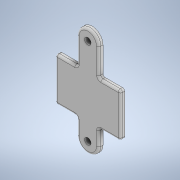
# Autodesk Inventor part: joy_mount_T
Saved by Autodesk Inventor 2021.4 (Build 254397000, 397)
## iProperties
Created: 2023-11-22
Part Number: joy_mount_T
Material: 一般
Document SubType Name: Modeling
Designer: ryusei
Density: 1 g/cm^3
Appearance: 既定
Author: ryusei
Autodesk Inventor part; units mm, degrees
ref_plane "YZ Plane" through (0, 0, 0) normal (1, 0, 0) x (0, 1, 0)
ref_plane "XZ Plane" through (0, 0, 0) normal (0, 1, 0) x (-1, 0, 0)
ref_plane "XY Plane" through (0, 0, 0) normal (0, 0, 1) x (1, 0, 0)
sketch "スケッチ1" plane through (0, 0, 0) normal (0, 0, 1) x (1, 0, 0)
  line L0 (-30, 20) -> (30, 20)
  line L1 (30, 20) -> (30, -20)
  line L2 (30, -20) -> (-30, -20)
  line L3 (-30, -20) -> (-30, 20)
  line L4 (-30, 20) -> (30, -20) construction
  line L5 (30, 20) -> (-30, -20) construction
  point P0 (0, 0)
  dimension "d0" = 60
  dimension "d1" = 40
  constraints: 12 end point, 2 midpoint, 2 parallel, 1 horizontal, 1 perpendicular
  measures "d0" distance of L1.end L2.end
  measures "d1" distance of L0.end L1.end
extrude "押し出し1" add sketch "スケッチ1" along normal blind 4
sketch "スケッチ2" plane through (0, 0, 4) normal (0, 0, 1) x (1, 0, 0)
  line L0 (-10, 55) -> (10, 55)
  line L1 (10, 55) -> (10, -45)
  line L2 (10, -45) -> (-10, -45)
  line L3 (-10, -45) -> (-10, 55)
  point P0 (0, 0)
  dimension "d4" = 20
  dimension "d5" = 100
  dimension "d6" = 10
  dimension "d7" = 55
  constraints: 8 end point, 2 parallel, 1 horizontal, 1 perpendicular
  measures "d4" distance of L1.end L2.end
  measures "d5" distance of L0.end L1.end
  measures "d6" distance from line of L3 point (0, 0)
  measures "d7" distance from line of point (0, 0) L0
extrude "押し出し2" add sketch "スケッチ2" against normal blind 4
fillet "フィレット1" radius 10 4 edges at (10, 55, 2) (-10, 55, 2) (10, -45, 2) (-10, -45, 2)
fillet "フィレット2" radius 2 22 edges at (10, 32.5001, 4) (-10, 32.5001, 4) (-7.0711, 52.0711, 4) (7.0711, 52.0711, 4) (20, 20, 4) (30, 0, 4) (20, -20, 4) (-7.0711, -42.0711, 4) (7.0711, -42.0711, 4) (-10, -27.5001, 4) (10, -27.5, 4) (-20, -20, 4) (-30, 0, 4) (-20, 20, 4) (-30, 20, 2) (-10, 20, 2) (-30, -20, 2) (-10, -20, 2) (10, -20, 2) (30, -20, 2) (30, 20, 2) (10, 20, 2)
sketch "スケッチ3" plane through (0, 0, 4) normal (0, 0, 1) x (1, 0, 0)
  arc A0 (10, 45) -> (-10, 45) centre (0, 45) ccw projected
  arc A1 (-10, -35) -> (10, -35) centre (0, -35) ccw projected
  point P0 (0, 0)
  dimension "d12" = 0
  dimension "d13" = 0
  measures "d12" distance of A0.centre point (0, 45)
  measures "d13" distance of A1.centre point (0, -35)
hole "穴1" at (0, -35, 4) at (0, 45, 4) direction (0, 0, -1) diameter 6 end through all
